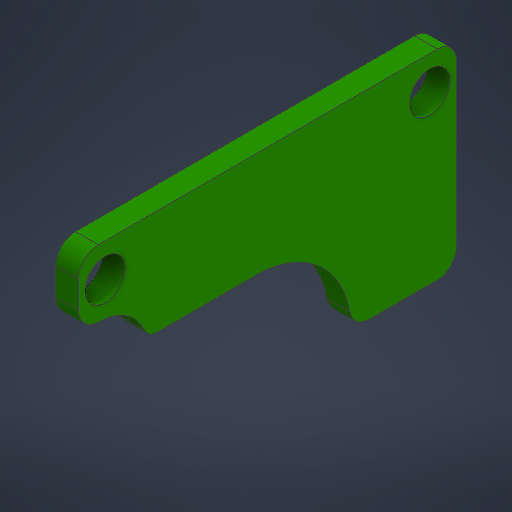
# Autodesk Inventor part: Lichtschrankenplatine
Saved by Autodesk Inventor 2025.2 (Build 292293000, 293)
## iProperties
Created: 2025-06-03
Part Number: Lichtschrankenplatine
Material: Generisch
Document SubType Name: Modeling
Designer: Faabs
Density: 1 g/cm^3
Appearance: Vorgabe
Author: Faabs
Autodesk Inventor part; units mm, degrees
ref_plane "YZ Plane" through (0, 0, 0) normal (1, 0, 0) x (0, 1, 0)
ref_plane "XZ Plane" through (0, 0, 0) normal (0, 1, 0) x (-1, 0, 0)
ref_plane "XY Plane" through (0, 0, 0) normal (0, 0, 1) x (1, 0, 0)
sketch "Skizze1" plane through (0, 0, 0) normal (1, 0, 0) x (0, 1, 0)
  line L0 (11.3779, 2.7501) -> (-5.6647, 2.75)
  arc A0 (-5.6647, 2.75) -> (-6.7086, 1.7062) centre (-5.6647, 1.7062) ccw
  line L1 (-6.7086, 1.7062) -> (-6.7086, 0.294)
  arc A1 (-6.7086, 0.294) -> (-5.6635, -0.7499) centre (-5.6647, 0.2939) ccw
  arc A2 (-3.2531, -2.3214) -> (-5.6635, -0.7499) centre (-5.6604, -3.3794) ccw
  arc A3 (-3.2531, -2.3214) -> (-2.5965, -2.75) centre (-2.5966, -2.0328) ccw
  line L2 (-2.5965, -2.75) -> (2.5966, -2.75)
  arc A4 (7.4824, -6.874) -> (2.5966, -2.75) centre (2.5966, -7.7061) ccw
  line L3 (8.4682, -7.7061) -> (12.0528, -7.7061)
  line L4 (13.0528, -6.7061) -> (13.0527, 1.7501)
  line L5 (12.0527, 2.7501) -> (11.3779, 2.7501)
  arc A5 (7.4824, -6.874) -> (8.4682, -7.7061) centre (8.4682, -6.7061) ccw
  arc A6 (12.0528, -7.7061) -> (13.0528, -6.7061) centre (12.0528, -6.7061) ccw
  arc A7 (13.0527, 1.7501) -> (12.0527, 2.7501) centre (12.0527, 1.7501) ccw
  line L6 (-6.7086, 1.0001) -> (-6.3086, 1.0001) construction
  circle A8 centre (-5.3086, 1.0001) radius 1.05
  circle A9 centre (11.6527, 1.0001) radius 1.05
  point P0 (0, 0)
  point P1 (13.0528, -7.7061)
  point P2 (0, 0)
  dimension "d9" = 5.5
  dimension "d10" = 1
  dimension "d11" = 0.4
  dimension "d12" = 2.1
  dimension "d13" = 1
  dimension "d16" = 2.1
  constraints: 16 point on circle, 14 end point, 10 centre point, 6 tangent, 2 equal radius, 2 point on line, 1 horizontal, 1 midpoint, 1 perpendicular
  measures "d9" distance between parallel lines of L0 L2
  measures "d10" radius of A5
  measures "d11" distance of L6.start L6.end
  measures "d12" diameter of A8
  measures "d13" distance of L6.end A8.centre
  measures "d16" diameter of A9
extrude "Extrusion1" add sketch "Skizze1" along normal blind 1.2
